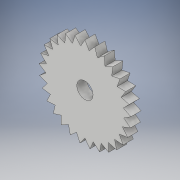
# Autodesk Inventor part: Backdrop Gear
Saved by Autodesk Inventor 2018 (Build 220112000, 112)
## iProperties
Created: 2018-12-13
Part Number: Backdrop Gear
Material: Generic
Document SubType Name: Modeling
Designer: F8PLTW
Density: 1 g/cm^3
Appearance: Default
Author: F8PLTW
Autodesk Inventor part; units mm, degrees
ref_plane "YZ Plane" through (0, 0, 0) normal (1, 0, 0) x (0, 1, 0)
ref_plane "XZ Plane" through (0, 0, 0) normal (0, 1, 0) x (-1, 0, 0)
ref_plane "XY Plane" through (0, 0, 0) normal (0, 0, 1) x (1, 0, 0)
sketch "Sketch1" plane through (0, 0, 0) normal (0, 0, 1) x (1, 0, 0)
  line L0 (-4.8577, 15.4767) -> (-7.8056, 15.4577)
  line L1 (-7.8056, 15.4577) -> (-6.3481, 18.0201)
  line L2 (-6.3481, 18.0201) -> (-4.8577, 15.4767)
  line L3 (-10.3164, 14.8652) -> (-9.4439, 17.6811)
  line L4 (-9.4439, 17.6811) -> (-7.4416, 15.5175)
  line L5 (-7.4416, 15.5175) -> (-10.3164, 14.8652)
  line L6 (-12.6412, 13.7469) -> (-12.3943, 16.6844)
  line L7 (-12.3943, 16.6844) -> (-9.9737, 15.0019)
  line L8 (-9.9737, 15.0019) -> (-12.6412, 13.7469)
  line L9 (-14.6712, 12.1549) -> (-15.0616, 15.0768)
  line L10 (-15.0616, 15.0768) -> (-12.3359, 13.954)
  line L11 (-12.3359, 13.954) -> (-14.6712, 12.1549)
  line L12 (-16.3115, 10.1637) -> (-17.3209, 12.9335)
  line L13 (-17.3209, 12.9335) -> (-14.4175, 12.4228)
  line L14 (-14.4175, 12.4228) -> (-16.3115, 10.1637)
  line L15 (-17.4854, 7.8665) -> (-19.0666, 10.3545)
  line L16 (-19.0666, 10.3545) -> (-16.1213, 10.4799)
  line L17 (-16.1213, 10.4799) -> (-17.4854, 7.8665)
  line L18 (-18.138, 5.3707) -> (-20.2171, 7.4605)
  line L19 (-20.2171, 7.4605) -> (-17.3677, 8.2162)
  line L20 (-17.3677, 8.2162) -> (-18.138, 5.3707)
  line L21 (-18.2388, 2.7929) -> (-20.7186, 4.3869)
  line L22 (-20.7186, 4.3869) -> (-18.0982, 5.7374)
  line L23 (-18.0982, 5.7374) -> (-18.2388, 2.7929)
  line L24 (-17.7832, 0.2536) -> (-20.5476, 1.2774)
  line L25 (-20.5476, 1.2774) -> (-18.2788, 3.1596)
  line L26 (-18.2788, 3.1596) -> (-17.7832, 0.2536)
  line L27 (-16.7923, -2.1282) -> (-19.7122, -1.7227)
  line L28 (-19.7122, -1.7227) -> (-17.901, 0.6032)
  line L29 (-17.901, 0.6032) -> (-16.7923, -2.1282)
  line L30 (-15.3125, -4.2414) -> (-18.2514, -4.4731)
  line L31 (-18.2514, -4.4731) -> (-16.9826, -1.8122)
  line L32 (-16.9826, -1.8122) -> (-15.3125, -4.2414)
  line L33 (-13.4131, -5.9871) -> (-16.2334, -6.8451)
  line L34 (-16.2334, -6.8451) -> (-15.5663, -3.9737)
  line L35 (-15.5663, -3.9737) -> (-13.4131, -5.9871)
  line L36 (-11.1828, -7.2837) -> (-13.7528, -8.7279)
  line L37 (-13.7528, -8.7279) -> (-13.7185, -5.7802)
  line L38 (-13.7185, -5.7802) -> (-11.1828, -7.2837)
  line L39 (-8.726, -8.0705) -> (-10.9253, -10.0334)
  line L40 (-10.9253, -10.0334) -> (-11.5256, -7.1472)
  line L41 (-11.5256, -7.1472) -> (-8.726, -8.0705)
  line L42 (-6.1574, -8.3107) -> (-7.8834, -10.7005)
  line L43 (-7.8834, -10.7005) -> (-9.09, -8.0109)
  line L44 (-9.09, -8.0109) -> (-6.1574, -8.3107)
  line L45 (-3.5972, -7.9932) -> (-4.7691, -10.6982)
  line L46 (-4.7691, -10.6982) -> (-6.5258, -8.3308)
  line L47 (-6.5258, -8.3308) -> (-3.5972, -7.9932)
  line L48 (-1.1652, -7.1327) -> (-1.7282, -10.0264)
  line L49 (-1.7282, -10.0264) -> (-3.9527, -8.092)
  line L50 (-3.9527, -8.092) -> (-1.1652, -7.1327)
  line L51 (1.025, -5.7695) -> (1.0972, -8.7166)
  line L52 (1.0972, -8.7166) -> (-1.4911, -7.3056)
  line L53 (-1.4911, -7.3056) -> (1.025, -5.7695)
  line L54 (2.871, -3.9674) -> (3.575, -6.83)
  line L55 (3.575, -6.83) -> (0.7439, -6.0084)
  line L56 (0.7439, -6.0084) -> (2.871, -3.9674)
  line L57 (4.2864, -1.8106) -> (5.5893, -4.4549)
  line L58 (5.5893, -4.4549) -> (2.6478, -4.2612)
  line L59 (2.6478, -4.2612) -> (4.2864, -1.8106)
  line L60 (5.205, 0.6001) -> (7.046, -1.7023)
  line L61 (7.046, -1.7023) -> (4.1315, -2.1455)
  line L62 (4.1315, -2.1455) -> (5.205, 0.6001)
  line L63 (5.584, 3.1519) -> (7.8768, 1.299)
  line L64 (7.8768, 1.299) -> (5.1258, 0.2398)
  line L65 (5.1258, 0.2398) -> (5.584, 3.1519)
  line L66 (5.4055, 5.7255) -> (8.0431, 4.4088)
  line L67 (8.0431, 4.4088) -> (5.5841, 2.7829)
  line L68 (5.5841, 2.7829) -> (5.4055, 5.7255)
  line L69 (4.678, 8.2005) -> (7.5369, 7.4817)
  line L70 (7.5369, 7.4817) -> (5.4849, 5.3652)
  line L71 (5.4849, 5.3652) -> (4.678, 8.2005)
  line L72 (3.4354, 10.4613) -> (6.382, 10.3739)
  line L73 (6.382, 10.3739) -> (4.833, 7.8657)
  line L74 (4.833, 7.8657) -> (3.4354, 10.4613)
  line L75 (1.7358, 12.4021) -> (4.6324, 12.9502)
  line L76 (4.6324, 12.9502) -> (3.6587, 10.1677)
  line L77 (3.6587, 10.1677) -> (1.7358, 12.4021)
  line L78 (-0.3412, 13.9322) -> (2.3698, 15.0901)
  line L79 (2.3698, 15.0901) -> (2.0171, 12.1634)
  line L80 (2.0171, 12.1634) -> (-0.3412, 13.9322)
  line L81 (-2.6986, 14.98) -> (-0.2999, 16.6936)
  line L82 (-0.2999, 16.6936) -> (-0.0152, 13.7595)
  line L83 (-0.0152, 13.7595) -> (-2.6986, 14.98)
  line L84 (-5.2261, 15.4966) -> (-3.2519, 17.6858)
  line L85 (-3.2519, 17.6858) -> (-2.3431, 14.8814)
  line L86 (-2.3431, 14.8814) -> (-5.2261, 15.4966)
  circle A0 centre (-6.3372, 3.6182) radius 11.9504
  point P0 (0, 0)
  point P1 (-6.3372, 16.3182)
  dimension "d3" = 360
  dimension "d10" = 2.9479
  constraints: 174 end point, 1 coincident, 185 other
  measures "d10" horizontal distance of L0.start L0.end
extrude "Extrusion1" add sketch "Sketch1" along normal blind 3.175
sketch "Sketch2" plane through (0, 0, 3.175) normal (0, 0, 1) x (1, 0, 0)
  line L0 (-6.3481, 18.0201) -> (-7.646, 15.7384) projected
  line L1 (-6.3464, -8.5725) -> (-6.3481, 18.0201) construction
  line L2 (-20.7186, 4.3869) -> (-18.5104, 2.9675) projected
  line L3 (8.0431, 4.4088) -> (5.6944, 5.5813) projected
  line L4 (-20.7186, 4.3869) -> (8.0431, 4.4088) construction
  circle A0 centre (-6.3378, 4.3979) radius 2.54
  point P0 (0, 0)
  dimension "d7" = 5.08
  constraints: 4 end point, 1 centre point, 1 midpoint
  measures "d7" diameter of A0
extrude "Extrusion2" cut sketch "Sketch2" against normal blind 3.175
body "Solid1"
